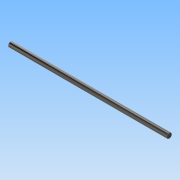
# Autodesk Inventor part: вал 12мм
Saved by Autodesk Inventor 2017 (Build 210142000, 142)
## iProperties
Part Number: вал 12мм
Material: Типовые
Document SubType Name: Modeling
Designer: Max
Mass: 40.6995 g
Surface Area: 137.646 cm^2
Volume: 40.6995 cm^3
Density: 1 g/cm^3
Appearance: Сталь — полированная
Author: Max
Autodesk Inventor part; units mm, degrees
ref_plane "YZ Plane" through (0, 0, 0) normal (1, 0, 0) x (0, 1, 0)
ref_plane "XZ Plane" through (0, 0, 0) normal (0, 1, 0) x (-1, 0, 0)
ref_plane "XY Plane" through (0, 0, 0) normal (0, 0, 1) x (1, 0, 0)
sketch "Эскиз1" plane through (0, 0, 0) normal (1, 0, 0) x (0, 1, 0)
  circle A0 centre (0, 0) radius 6
  dimension "d0" = 12
  constraints: 1 centre point, 1 coincident
  measures "d0" diameter of A0
extrude "Выдавливание1" add sketch "Эскиз1" along normal blind 360
fillet "Сопряжение1" radius 1 2 edges at (360, -6, 0) (0, -6, 0)
